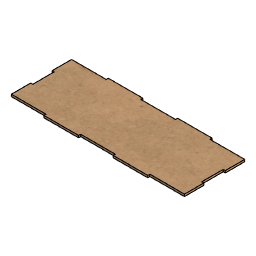
Step top v7 (Autodesk Fusion 360 design; units mm, degrees)
Autodesk Fusion 360 part; units mm, degrees
sketch "Sketch1" plane through (0, 0, 0) normal (0, 0, 1) x (1, 0, 0)
  line L0 (125, 46.5) -> (-125, 46.5)
  line L1 (-125, 46.5) -> (-125, -46.5)
  line L2 (-125, -46.5) -> (125, -46.5)
  line L3 (125, -46.5) -> (125, 46.5)
  line L4 (125, 46.5) -> (-125, -46.5) construction
  line L5 (-125, 46.5) -> (125, -46.5) construction
  line L6 (-125, 46.5) -> (-75, 46.5)
  line L7 (-75, 46.5) -> (-75, 43.5)
  line L8 (-75, 43.5) -> (-125, 43.5)
  line L9 (-125, 43.5) -> (-125, 46.5)
  line L10 (25, 43.5) -> (-25, 43.5)
  line L11 (-25, 46.5) -> (25, 46.5)
  line L12 (25, 46.5) -> (25, 43.5)
  line L13 (-25, 43.5) -> (-25, 46.5)
  line L14 (125, 43.5) -> (75, 43.5)
  line L15 (75, 46.5) -> (125, 46.5)
  line L16 (125, 46.5) -> (125, 43.5)
  line L17 (75, 43.5) -> (75, 46.5)
  line L18 (-75, -46.5) -> (-125, -46.5)
  line L19 (-125, -43.5) -> (-75, -43.5)
  line L20 (-75, -43.5) -> (-75, -46.5)
  line L21 (-125, -46.5) -> (-125, -43.5)
  line L22 (25, -46.5) -> (-25, -46.5)
  line L23 (-25, -43.5) -> (25, -43.5)
  line L24 (25, -43.5) -> (25, -46.5)
  line L25 (-25, -46.5) -> (-25, -43.5)
  line L26 (125, -46.5) -> (75, -46.5)
  line L27 (75, -43.5) -> (125, -43.5)
  line L28 (125, -43.5) -> (125, -46.5)
  line L29 (75, -46.5) -> (75, -43.5)
  dimension "d1" = 250
  dimension "d2" = 93
  dimension "d13" = 50
  dimension "d14" = 3
  dimension "d17" = 200
  dimension "d18" = -90
  constraint horizontal L0
  constraint perpendicular L0 L1
  constraint parallel L0 L2
  constraint parallel L1 L3
  constraint coincident L4 origin
  constraint coincident L5 origin
  constraint horizontal L6
  constraint vertical L7
  constraint horizontal L8
  constraint vertical L9
  measures "d1" distance of L1.end L2.end
  measures "d2" distance of L0.end L1.end
  measures "d13" distance of L0.end L6.end
  measures "d14" distance of L0.end L8.end
extrude "Extrude3" add sketch "Sketch1" along normal blind 3 contours L0 L1 L2 L3 L7 L8 L10 L12 L13 L14 L17 L19 L20 L23 L24 L25 L27 L29
sketch "Sketch3" plane through (0, 0, 3) normal (0, 0, 1) x (-1, 0, 0)
  line L0 (-75, 46.5) -> (-75, 43.5)
  line L1 (-75, 43.5) -> (-125, 43.5)
  line L2 (-125, 43.5) -> (-125, -43.5)
  line L3 (-125, -43.5) -> (-75, -43.5)
  line L4 (-75, -43.5) -> (-75, -46.5)
  line L5 (-75, -46.5) -> (-25, -46.5)
  line L6 (-25, -46.5) -> (-25, -43.5)
  line L7 (-25, -43.5) -> (25, -43.5)
  line L8 (25, -43.5) -> (25, -46.5)
  line L9 (25, -46.5) -> (75, -46.5)
  line L10 (75, -46.5) -> (75, -43.5)
  line L11 (75, -43.5) -> (125, -43.5)
  line L12 (125, -43.5) -> (125, 43.5)
  line L13 (125, 43.5) -> (75, 43.5)
  line L14 (75, 43.5) -> (75, 46.5)
  line L15 (75, 46.5) -> (25, 46.5)
  line L16 (25, 46.5) -> (25, 43.5)
  line L17 (25, 43.5) -> (-25, 43.5)
  line L18 (-25, 43.5) -> (-25, 46.5)
  line L19 (-25, 46.5) -> (-75, 46.5)
  line L20 (-121.1564, -43.5) -> (-121.1564, -15.5) construction
  line L21 (-121.1564, 43.5) -> (-121.1564, 15.5) construction
  line L22 (-125, -15.5) -> (-122, -15.5)
  line L23 (-122, -15.5) -> (-122, 15.5)
  line L24 (-122, 15.5) -> (-125, 15.5)
  line L25 (-125, 15.5) -> (-125, -15.5)
  dimension "d21" = 28
  dimension "d22" = 28
  dimension "d23" = 3
  dimension "d24" = 31
  constraint coincident L3 L20.start
  constraint perpendicular L3 L20
  constraint coincident L1 L21.start
  constraint perpendicular L1 L21
  constraint horizontal L22
  constraint vertical L23
  constraint horizontal L24
  constraint vertical L25
  constraint coincident L2 L22.start
  measures "d21" distance of L20.start L20.end
  measures "d22" distance of L21.start L21.end
  measures "d23" distance of L22.start L22.end
  measures "d24" distance of L22.start L24.end
extrude "Extrude4" cut sketch "Sketch3" against normal blind 6 contours L2 L22 L23 L24 L25
mirror "Mirror1" about plane through (0, 0, 0) normal (1, 0, 0) of "Extrude4"
sketch "Sketch4" plane through (0, 0, 3) normal (0, 0, 1) x (-1, 0, 0)
  line L0 (122, 15.5) -> (125, 15.5)
  line L1 (125, 15.5) -> (125, 43.5)
  line L2 (125, 43.5) -> (75, 43.5)
  line L3 (75, 43.5) -> (75, 46.5)
  line L4 (75, 46.5) -> (25, 46.5)
  line L5 (25, 46.5) -> (25, 43.5)
  line L6 (25, 43.5) -> (-25, 43.5)
  line L7 (-25, 43.5) -> (-25, 46.5)
  line L8 (-25, 46.5) -> (-75, 46.5)
  line L9 (-75, 46.5) -> (-75, 43.5)
  line L10 (-75, 43.5) -> (-125, 43.5)
  line L11 (-125, 43.5) -> (-125, 15.5)
  line L12 (-125, 15.5) -> (-122, 15.5)
  line L13 (-122, 15.5) -> (-122, -15.5)
  line L14 (-122, -15.5) -> (-125, -15.5)
  line L15 (-125, -15.5) -> (-125, -43.5)
  line L16 (-125, -43.5) -> (-75, -43.5)
  line L17 (-75, -43.5) -> (-75, -46.5)
  line L18 (-75, -46.5) -> (-25, -46.5)
  line L19 (-25, -46.5) -> (-25, -43.5)
  line L20 (-25, -43.5) -> (25, -43.5)
  line L21 (25, -43.5) -> (25, -46.5)
  line L22 (25, -46.5) -> (75, -46.5)
  line L23 (75, -46.5) -> (75, -43.5)
  line L24 (75, -43.5) -> (125, -43.5)
  line L25 (125, -43.5) -> (125, -15.5)
  line L26 (125, -15.5) -> (122, -15.5)
  line L27 (122, -15.5) -> (122, 15.5)
